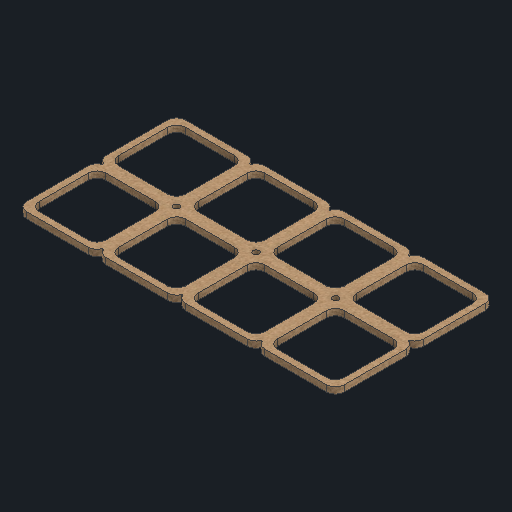
# Autodesk Inventor part: ProductsStoringGrid
Saved by Autodesk Inventor 2027.1 (Build 311270010, 270A)
## iProperties
Created: 2026-09-29
Part Number: ProductsStoringGrid
Material: MDF Medium Density Fiberboard
Document SubType Name: Modeling
Designer: SDS Scholar
Density: 0.8 g/cm^3
Appearance: Cardboard - Corrugated
Author: SDS Scholar
Autodesk Inventor part; units mm, degrees
ref_plane "YZ Plane" through (0, 0, 0) normal (1, 0, 0) x (0, 1, 0)
ref_plane "XZ Plane" through (0, 0, 0) normal (0, 1, 0) x (-1, 0, 0)
ref_plane "XY Plane" through (0, 0, 0) normal (0, 0, 1) x (1, 0, 0)
sketch "Sketch1" plane through (0, 0, 0) normal (0, 1, 0) x (-1, 0, 0)
  line L0 (114, 58) -> (75, 58)
  line L1 (68, 51) -> (68, 12)
  line L2 (75, 5) -> (114, 5)
  line L3 (121, 12) -> (121, 51)
  line L4 (119, 63) -> (70, 63)
  line L5 (63, 56) -> (63, 7)
  line L6 (70, 0) -> (119, 0)
  line L7 (126, 7) -> (126, 56)
  arc A0 (126, 56) -> (119, 63) centre (119, 56) ccw
  arc A1 (119, 0) -> (126, 7) centre (119, 7) ccw
  arc A2 (114, 5) -> (121, 12) centre (114, 12) ccw
  arc A3 (121, 51) -> (114, 58) centre (114, 51) ccw
  arc A4 (75, 58) -> (68, 51) centre (75, 51) ccw
  arc A5 (68, 12) -> (75, 5) centre (75, 12) ccw
  arc A6 (63, 7) -> (70, 0) centre (70, 7) ccw
  arc A7 (70, 63) -> (63, 56) centre (70, 56) ccw
  line L8 (0, 100) -> (0, -100) construction
  line L9 (100, 0) -> (-100, 0) construction
  line L10 (68, -12) -> (68, -51)
  line L11 (75, -58) -> (114, -58)
  line L12 (63, -7) -> (63, -56)
  arc A8 (75, -5) -> (68, -12) centre (75, -12) ccw
  line L13 (70, -63) -> (119, -63)
  arc A9 (70, 0) -> (63, -7) centre (70, -7) ccw
  line L14 (114, -5) -> (75, -5)
  line L15 (119, 0) -> (70, 0)
  arc A10 (126, -7) -> (119, 0) centre (119, -7) ccw
  arc A11 (63, -56) -> (70, -63) centre (70, -56) ccw
  arc A12 (68, -51) -> (75, -58) centre (75, -51) ccw
  line L16 (121, -51) -> (121, -12)
  line L17 (126, -56) -> (126, -7)
  arc A13 (121, -12) -> (114, -5) centre (114, -12) ccw
  arc A14 (114, -58) -> (121, -51) centre (114, -51) ccw
  arc A15 (119, -63) -> (126, -56) centre (119, -56) ccw
  line L18 (12, 5) -> (51, 5)
  line L19 (58, 12) -> (58, 51)
  line L20 (7, 0) -> (56, 0)
  line L21 (63, 7) -> (63, 56)
  arc A16 (5, 12) -> (12, 5) centre (12, 12) ccw
  line L22 (0, 56) -> (0, 7)
  line L23 (5, 51) -> (5, 12)
  arc A17 (58, 51) -> (51, 58) centre (51, 51) ccw
  arc A18 (63, 56) -> (56, 63) centre (56, 56) ccw
  line L24 (51, 58) -> (12, 58)
  line L25 (56, 63) -> (7, 63)
  arc A19 (51, 5) -> (58, 12) centre (51, 12) ccw
  arc A20 (7, 63) -> (0, 56) centre (7, 56) ccw
  arc A21 (12, 58) -> (5, 51) centre (12, 51) ccw
  arc A22 (56, 0) -> (63, 7) centre (56, 7) ccw
  arc A23 (0, 7) -> (7, 0) centre (7, 7) ccw
  line L26 (5, -12) -> (5, -51)
  line L27 (0, -7) -> (0, -56)
  arc A24 (5, -51) -> (12, -58) centre (12, -51) ccw
  arc A25 (0, -56) -> (7, -63) centre (7, -56) ccw
  line L28 (51, -5) -> (12, -5)
  line L29 (56, 0) -> (7, 0)
  arc A26 (58, -12) -> (51, -5) centre (51, -12) ccw
  arc A27 (63, -7) -> (56, 0) centre (56, -7) ccw
  line L30 (58, -51) -> (58, -12)
  line L31 (63, -56) -> (63, -7)
  line L32 (12, -58) -> (51, -58)
  line L33 (7, -63) -> (56, -63)
  arc A28 (51, -58) -> (58, -51) centre (51, -51) ccw
  arc A29 (12, -5) -> (5, -12) centre (12, -12) ccw
  arc A30 (56, -63) -> (63, -56) centre (56, -56) ccw
  arc A31 (7, 0) -> (0, -7) centre (7, -7) ccw
  line L34 (-51, 5) -> (-12, 5)
  line L35 (-5, 12) -> (-5, 51)
  line L36 (-56, 0) -> (-7, 0)
  line L37 (0, 7) -> (0, 56)
  arc A32 (-58, 12) -> (-51, 5) centre (-51, 12) ccw
  line L38 (-63, 56) -> (-63, 7)
  line L39 (-58, 51) -> (-58, 12)
  arc A33 (-5, 51) -> (-12, 58) centre (-12, 51) ccw
  arc A34 (0, 56) -> (-7, 63) centre (-7, 56) ccw
  line L40 (-12, 58) -> (-51, 58)
  line L41 (-7, 63) -> (-56, 63)
  arc A35 (-12, 5) -> (-5, 12) centre (-12, 12) ccw
  arc A36 (-56, 63) -> (-63, 56) centre (-56, 56) ccw
  arc A37 (-51, 58) -> (-58, 51) centre (-51, 51) ccw
  arc A38 (-7, 0) -> (0, 7) centre (-7, 7) ccw
  arc A39 (-63, 7) -> (-56, 0) centre (-56, 7) ccw
  line L42 (-58, -12) -> (-58, -51)
  line L43 (-63, -7) -> (-63, -56)
  arc A40 (-58, -51) -> (-51, -58) centre (-51, -51) ccw
  arc A41 (-63, -56) -> (-56, -63) centre (-56, -56) ccw
  line L44 (-12, -5) -> (-51, -5)
  line L45 (-7, 0) -> (-56, 0)
  arc A42 (-5, -12) -> (-12, -5) centre (-12, -12) ccw
  arc A43 (0, -7) -> (-7, 0) centre (-7, -7) ccw
  line L46 (-5, -51) -> (-5, -12)
  line L47 (0, -56) -> (0, -7)
  line L48 (-51, -58) -> (-12, -58)
  line L49 (-56, -63) -> (-7, -63)
  arc A44 (-12, -58) -> (-5, -51) centre (-12, -51) ccw
  arc A45 (-51, -5) -> (-58, -12) centre (-51, -12) ccw
  arc A46 (-7, -63) -> (0, -56) centre (-7, -56) ccw
  arc A47 (-56, 0) -> (-63, -7) centre (-56, -7) ccw
  line L50 (-114, 5) -> (-75, 5)
  line L51 (-68, 12) -> (-68, 51)
  line L52 (-119, 0) -> (-70, 0)
  line L53 (-63, 7) -> (-63, 56)
  arc A48 (-121, 12) -> (-114, 5) centre (-114, 12) ccw
  line L54 (-126, 56) -> (-126, 7)
  line L55 (-121, 51) -> (-121, 12)
  arc A49 (-68, 51) -> (-75, 58) centre (-75, 51) ccw
  arc A50 (-63, 56) -> (-70, 63) centre (-70, 56) ccw
  line L56 (-75, 58) -> (-114, 58)
  line L57 (-70, 63) -> (-119, 63)
  arc A51 (-75, 5) -> (-68, 12) centre (-75, 12) ccw
  arc A52 (-119, 63) -> (-126, 56) centre (-119, 56) ccw
  arc A53 (-114, 58) -> (-121, 51) centre (-114, 51) ccw
  arc A54 (-70, 0) -> (-63, 7) centre (-70, 7) ccw
  arc A55 (-126, 7) -> (-119, 0) centre (-119, 7) ccw
  line L58 (-121, -12) -> (-121, -51)
  line L59 (-126, -7) -> (-126, -56)
  arc A56 (-121, -51) -> (-114, -58) centre (-114, -51) ccw
  arc A57 (-126, -56) -> (-119, -63) centre (-119, -56) ccw
  line L60 (-75, -5) -> (-114, -5)
  line L61 (-70, 0) -> (-119, 0)
  arc A58 (-68, -12) -> (-75, -5) centre (-75, -12) ccw
  arc A59 (-63, -7) -> (-70, 0) centre (-70, -7) ccw
  line L62 (-68, -51) -> (-68, -12)
  line L63 (-63, -56) -> (-63, -7)
  line L64 (-114, -58) -> (-75, -58)
  line L65 (-119, -63) -> (-70, -63)
  arc A60 (-75, -58) -> (-68, -51) centre (-75, -51) ccw
  arc A61 (-114, -5) -> (-121, -12) centre (-114, -12) ccw
  arc A62 (-70, -63) -> (-63, -56) centre (-70, -56) ccw
  arc A63 (-119, 0) -> (-126, -7) centre (-119, -7) ccw
  circle A64 centre (63, 0) radius 2.5
  circle A65 centre (0, 0) radius 2.5
  circle A66 centre (-63, 0) radius 2.5
  point P0 (121, 58)
  point P1 (68, 5)
  point P2 (121, 5)
  point P3 (68, -58)
  point P4 (121, -58)
  point P5 (121, -5)
  point P6 (94.5, 0)
  point P7 (58, 5)
  point P8 (5, 5)
  point P9 (58, 58)
  point P10 (5, -58)
  point P11 (58, -5)
  point P12 (31.5, 0)
  point P13 (58, -58)
  point P14 (-5, 5)
  point P15 (-58, 5)
  point P16 (-5, 58)
  point P17 (-58, -58)
  point P18 (-5, -5)
  point P19 (-31.5, 0)
  point P20 (-5, -58)
  point P21 (-68, 5)
  point P22 (-121, 5)
  point P23 (-68, 58)
  point P24 (-121, -58)
  point P25 (-68, -5)
  point P26 (-94.5, 0)
  point P27 (-68, -58)
  point P28 (0, -31.5)
  point P29 (63, -31.5)
  point P30 (-63, -31.5)
  point P31 (119, 0)
  point P32 (63, 56)
  point P33 (0, 56)
  point P34 (-63, 56)
  point P35 (-119, 0)
  point P36 (-63, -56)
  point P37 (0, -56)
  point P38 (63, -56)
  point P39 (-63, 56)
  point P40 (-63, 7)
  point P41 (0, 56)
  point P42 (0, 7)
  point P43 (63, 7)
  point P44 (63, 56)
  point P45 (63, -7)
  point P46 (63, -56)
  point P47 (0, -7)
  point P48 (0, -56)
  point P49 (-63, -7)
  dimension "d0" = 53
  dimension "d1" = 53
  dimension "d2" = 5
  dimension "d3" = 7
  dimension "d4" = 200
  dimension "d6" = 200
  dimension "d9" = 63
  dimension "d19" = 63
  dimension "d23" = 5
  dimension "d24" = 5
  dimension "d25" = 5
  constraints: 132 end point, 128 point on circle, 67 centre point, 50 point on line, 16 tangent, 7 equal radius, 6 midpoint, 4 parallel, 3 horizontal, 3 vertical alignment, 2 coincident, 2 perpendicular, 2 vertical, 1 horizontal alignment, 307 other
  measures "d0" distance of point (68, 5) point (121, 5)
  measures "d1" distance of point (121, 5) point (121, 58)
  measures "d2" distance between parallel lines of L3 L7
  measures "d3" radius of A0
  measures "d4" distance of L8.start L8.end
  measures "d6" distance of L9.start L9.end
  measures "d9" distance of L1.end L10.end
  measures "d19" distance of L2.start L18.start
  measures "d23" diameter of A64
  measures "d24" diameter of A65
  measures "d25" diameter of A66
extrude "Extrusion1" add sketch "Sketch1" along normal blind 5
fillet "Fillet1" radius 0.5 8 edges at (119, 2.5, 0) (63, 2.5, 56) (0, 2.5, 56) (-63, 2.5, 56) (-119, 2.5, 0) (-63, 2.5, -56) (0, 2.5, -56) (63, 2.5, -56)
equation "\"d0\" = Product_dia + GridProcutClearance"
equation "\"d1\" = Product_dia + GridProcutClearance"
equation "\"d2\" = GridBorderThickness"
equation "\"d3\" = GridBorderFillets"
equation "\"d9\" = GridTotalSize"
equation "\"d19\" = GridTotalSize"
equation "\"Product_dia\" = 50"
equation "\"GridBorderThickness\" = 5"
equation "\"GridBorderFillets\" = 7"
equation "\"GridTotalSize\" = 63"
equation "\"GridProcutClearance\" = 3"
equation "\"BaseTotalWidth\" = 412"
equation "\"BaseTotalLength\" = 624"
equation "\"DistanceBetweenGrid\" = 5"
equation "\"WorkspaceLength\" = 395"
equation "\"WorkspaceWidth\" = 332"
equation "\"AxesBaseFillet\" = 15"
equation "\"Zaxis\" = 127"
body "Solid1"
